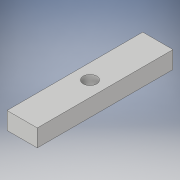
# Autodesk Inventor part: BeltMount
Saved by Autodesk Inventor 2019 (Build 230136000, 136)
## iProperties
Created: 2019-01-17
Part Number: BeltMount
Material: Generic
Document SubType Name: Modeling
Designer: nxgam
Density: 1 g/cm^3
Appearance: Default
Author: nxgam
Autodesk Inventor part; units mm, degrees
ref_plane "YZ Plane" through (0, 0, 0) normal (1, 0, 0) x (0, 1, 0)
ref_plane "XZ Plane" through (0, 0, 0) normal (0, 1, 0) x (-1, 0, 0)
ref_plane "XY Plane" through (0, 0, 0) normal (0, 0, 1) x (1, 0, 0)
sketch "Sketch1" plane through (0, 0, 0) normal (0, 1, 0) x (-1, 0, 0)
  line L0 (-4.445, 19.939) -> (4.445, 19.939)
  line L1 (4.445, 19.939) -> (4.445, -19.939)
  line L2 (4.445, -19.939) -> (-4.445, -19.939)
  line L3 (-4.445, -19.939) -> (-4.445, 19.939)
  line L4 (-4.445, 19.939) -> (4.445, -19.939) construction
  line L5 (4.445, 19.939) -> (-4.445, -19.939) construction
  circle A0 centre (0, 0) radius 2
  dimension "d0" = 8.89
  dimension "d1" = 39.878
  dimension "d2" = 4
  constraints: 12 end point, 2 midpoint, 2 parallel, 1 centre point, 1 coincident, 1 horizontal, 1 perpendicular
  measures "d0" distance of L1.end L2.end
  measures "d1" distance of L0.end L1.end
  measures "d2" diameter of A0
extrude "Extrusion1" add sketch "Sketch1" along normal blind 5.08
body "Solid1"
